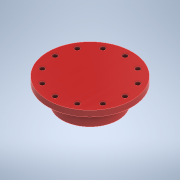
# Autodesk Inventor part: topAttachementForPvcPipe
Saved by Autodesk Inventor 2022.2 (Build 262287000, 287)
## iProperties
Created: 2021-10-20
Part Number: topAttachementForPvcPipe
Material: PC/ABS Plastic
Document SubType Name: Modeling
Designer: robst
Density: 0.357273 g/cm^3
Appearance: Red
Author: robst
Autodesk Inventor part; units mm, degrees
ref_plane "YZ Plane" through (0, 0, 0) normal (1, 0, 0) x (0, 1, 0)
ref_plane "XZ Plane" through (0, 0, 0) normal (0, 1, 0) x (-1, 0, 0)
ref_plane "XY Plane" through (0, 0, 0) normal (0, 0, 1) x (1, 0, 0)
sketch "Sketch51" plane through (0, 0, 0) normal (0, 1, 0) x (-1, 0, 0)
  circle A0 centre (0, 0) radius 57.15
  dimension "d242" = 114.3
  constraints: 1 centre point, 1 coincident
  measures "d242" diameter of A0
extrude "Extrusion26" add sketch "Sketch51" against normal blind 8
sketch "Sketch58" plane through (0, 0, 0) normal (0, 1, 0) x (1, 0, 0)
  circle A0 centre (0, 0) radius 31.4309 construction
  point P0 (0, 47.625)
  point P1 (-23.8125, 41.2445)
  point P2 (-41.2445, 23.8125)
  point P3 (-47.625, 0)
  point P4 (-41.2445, -23.8125)
  point P5 (-23.8125, -41.2445)
  point P6 (0, -47.625)
  point P7 (23.8125, -41.2445)
  point P8 (41.2445, -23.8125)
  point P9 (47.625, 0)
  point P10 (41.2445, 23.8125)
  point P11 (23.8125, 41.2445)
  dimension "d294" = 47.625
  dimension "d297" = 360
  constraints: 1 centre point, 13 other
  measures "d294" distance of point (0, 47.625) point (0, 0)
hole "Hole9" at (0, 0, -47.625) at (-23.8125, 0, -41.2445) at (-41.2445, 0, -23.8125) at (-47.625, 0, 0) at (-41.2445, 0, 23.8125) at (-23.8125, 0, 41.2445) at (0, 0, 47.625) at (23.8125, 0, 41.2445) at (41.2445, 0, 23.8125) at (47.625, 0, 0) at (41.2445, 0, -23.8125) at (23.8125, 0, -41.2445) direction (0, -1, 0) diameter 5.105 end through all counterbore diameter 6.3754 counterbore depth 9.525 clearance for "Hex Machine Screw" size "#10" standard "Ansi Unified Screw Threads"
sketch "Sketch59" plane through (0, -8, 0) normal (0, -1, 0) x (1, 0, 0)
  circle A0 centre (0, 0) radius 38.1
  circle A1 centre (0, 0) radius 28.575
  dimension "d306" = 76.2
  dimension "d307" = 9.525
  constraints: 2 centre point, 2 coincident
  measures "d306" diameter of A0
  measures "d307" radial gap between concentric circles of A1 A0
extrude "Extrusion29" add sketch "Sketch59" along normal blind 25
equation "\"d242\" = outsideDiameterOfPart"
equation "\"d243\" = wallThickness"
equation "\"d306\" = insideDiameterOfPipe"
equation "\"wallThickness\" = 8"
equation "\"twoByFourWidth\" = 40.64"
equation "\"twoByFourDepth\" = 84.1375"
equation "\"azimuth\" = 55deg"
equation "\"elevationOfTwoByFour\" = 20deg"
equation "\"depthOfExtrusionForMatingToLowerHalf\" = 12.5"
equation "\"depthForWasherForMatingToCase\" = 14"
equation "\"pvc2InchPipeInsideDiameter\" = 52.5018"
equation "\"pvc2InchPipeOutsideDiameter\" = 60.325"
equation "\"pvcPipeInsertDepth\" = 25"
equation "\"outsideDiameterOfPipe\" = 88.9"
equation "\"insideDiameterOfPipe\" = 76.2"
equation "\"outsideDiameterOfPart\" = 114.3"
body "Solid4"
